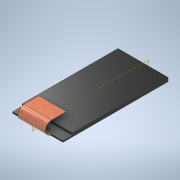
# Autodesk Inventor part: Display_1.3
Saved by Autodesk Inventor 2020 (Build 240168000, 168)
## iProperties
Created: 2022-06-10
Part Number: Display_1.3
Material: Типовые
Document SubType Name: Modeling
Designer: NoName
Density: 1 g/cm^3
Appearance: По умолчанию
Author: NoName
Autodesk Inventor part; units mm, degrees
ref_plane "YZ Plane" through (0, 0, 0) normal (1, 0, 0) x (0, 1, 0)
ref_plane "XZ Plane" through (0, 0, 0) normal (0, 1, 0) x (-1, 0, 0)
ref_plane "XY Plane" through (0, 0, 0) normal (0, 0, 1) x (1, 0, 0)
sketch "Эскиз1" plane through (0, 0, 0) normal (0, 1, 0) x (-1, 0, 0)
  line L0 (0, 0) -> (-17.1, 0)
  line L1 (-17.1, 0) -> (-17.1, -35.8)
  line L2 (-17.1, -35.8) -> (0, -35.8)
  line L3 (0, -35.8) -> (0, 0)
  dimension "d0" = 17.1
  dimension "d1" = 35.8
  constraints: 8 end point, 2 parallel, 1 horizontal, 1 perpendicular
  measures "d0" distance between parallel lines of L1 L3
  measures "d1" distance between parallel lines of L0 L2
extrude "Выдавливание1" add sketch "Эскиз1" along normal blind 0.5
sketch "Эскиз2" plane through (0, 0.5, 0) normal (0, 1, 0) x (1, 0, 0)
  line L0 (0, 35.8) -> (0, 0) projected
  line L1 (17.1, 0) -> (17.1, 35.8) projected
  line L2 (0, 35.8) -> (17.1, 35.8)
  line L3 (17.1, 35.8) -> (17.1, 3.2)
  line L4 (17.1, 3.2) -> (0, 3.2)
  line L5 (0, 3.2) -> (0, 35.8)
  point P0 (0, 3.2)
  dimension "d4" = 32.6
  constraints: 8 end point, 2 parallel, 1 horizontal, 1 perpendicular, 1 point on line
  measures "d4" distance between parallel lines of L2 L4
extrude "Выдавливание2" add sketch "Эскиз2" along normal blind 0.7
sketch "Эскиз3" plane through (0, 0, 0) normal (0, -1, 0) x (1, 0, 0)
  line L0 (0, -35.8) -> (0, -3.2) projected
  line L1 (0, -3.2) -> (17.1, -3.2) projected
  line L2 (17.1, -3.2) -> (17.1, -35.8) projected
  line L3 (17.1, -35.8) -> (0, -35.8) projected
  line L4 (15.9, -34.2) -> (1.2, -34.2)
  line L5 (1.2, -34.2) -> (1.2, -4.8)
  line L6 (1.2, -4.8) -> (15.9, -4.8)
  line L7 (15.9, -4.8) -> (15.9, -34.2)
  point P0 (0, 0)
  point P1 (8.55, -34.2)
  point P2 (8.55, -35.8)
  point P3 (15.9, -19.5)
  point P4 (17.1, -19.5)
  dimension "d7" = 29.4
  dimension "d8" = 14.7
  constraints: 8 end point, 4 midpoint, 2 parallel, 1 horizontal, 1 horizontal alignment, 1 perpendicular, 1 vertical alignment
  measures "d7" distance of L6.end L4.start
  measures "d8" distance between parallel lines of L5 L7
extrude "Выдавливание3" cut sketch "Эскиз3" against normal blind 0.01 contours L4 L5 L6 L7
ref_plane "РабПлоскость1" through (8.55, 0, 0) normal (1, 0, 0) x (0, 0, -1)
sketch "Эскиз4" plane through (8.55, 0, 0) normal (1, 0, 0) x (0, 0, -1)
  line L0 (0, 0) -> (0, 0.5) projected
  arc A0 (0, 4.5) -> (0, 0.5) centre (0, 2.5) ccw
  arc A1 (0, 4.6) -> (0, 0.4) centre (0, 2.5) ccw
  line L1 (0, 4.5) -> (5.0168, 4.5)
  line L2 (5.0168, 4.5) -> (5.0168, 4.6)
  line L3 (5.0168, 4.6) -> (0, 4.6)
  dimension "d11" = 0.1
  dimension "d12" = 2
  dimension "d13" = 5.0168
  constraints: 6 end point, 4 point on circle, 4 vertical alignment, 2 centre point, 2 perpendicular, 2 point on line, 1 coincident, 1 horizontal
  measures "d11" radial gap between concentric circles of A1 A0
  measures "d12" radius of A0
  measures "d13" distance of L3.end L2.end
extrude "Выдавливание4" add sketch "Эскиз4" along normal mid plane 9.3
